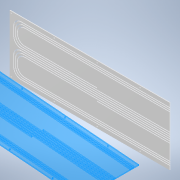
# Autodesk Inventor part: Part2
Saved by Autodesk Inventor 2021 (Build 250183000, 183)
## iProperties
Created: 2022-01-19
Part Number: Part2
Material: PVC-Piping
Document SubType Name: Modeling
Designer: avan411
Density: 1.4 g/cm^3
Appearance: Smooth - White
Author: avan411
Autodesk Inventor part; units mm, degrees
ref_plane "YZ Plane" through (0, 0, 0) normal (1, 0, 0) x (0, 1, 0)
ref_plane "XZ Plane" through (0, 0, 0) normal (0, 1, 0) x (-1, 0, 0)
ref_plane "XY Plane" through (0, 0, 0) normal (0, 0, 1) x (1, 0, 0)
sketch "Sketch1" plane through (0, 0, 0) normal (0, 0, 1) x (1, 0, 0)
  line L0 (97.5839, -88.8585) -> (97.5839, -84.5585) projected
  line L1 (97.5839, -88.8585) -> (532.0839, -88.8585) projected
  arc A0 (572.9339, -129.7085) -> (532.0839, -88.8585) centre (532.0839, -129.7085) ccw projected
  line L2 (572.9339, -129.7085) -> (572.9339, -137.9085) projected
  arc A1 (532.0839, -178.7585) -> (572.9339, -137.9085) centre (532.0839, -137.9085) ccw projected
  line L3 (532.0839, -178.7585) -> (-336.9161, -178.7585) projected
  arc A2 (-377.7661, -137.9085) -> (-336.9161, -178.7585) centre (-336.9161, -137.9085) ccw projected
  line L4 (-377.7661, -137.9085) -> (-377.7661, -118.2752) projected
  arc A3 (-336.9161, -77.4252) -> (-377.7661, -118.2752) centre (-336.9161, -118.2752) ccw projected
  line L5 (-336.9161, -77.4252) -> (543.3339, -77.4252) projected
  arc A4 (584.1839, -118.2752) -> (543.3339, -77.4252) centre (543.3339, -118.2752) ccw projected
  line L6 (584.1839, -118.2752) -> (584.1839, -148.6585) projected
  arc A5 (543.3339, -189.5085) -> (584.1839, -148.6585) centre (543.3339, -148.6585) ccw projected
  line L7 (543.3339, -189.5085) -> (-348.1661, -189.5085) projected
  arc A6 (-389.0161, -148.6585) -> (-348.1661, -189.5085) centre (-348.1661, -148.6585) ccw projected
  line L8 (-389.0161, -148.6585) -> (-389.0161, -106.8419) projected
  arc A7 (-348.1661, -65.9919) -> (-389.0161, -106.8419) centre (-348.1661, -106.8419) ccw projected
  line L9 (-348.1661, -65.9919) -> (554.5839, -65.9919) projected
  arc A8 (595.4339, -106.8419) -> (554.5839, -65.9919) centre (554.5839, -106.8419) ccw projected
  line L10 (595.4339, -106.8419) -> (595.4339, -159.4085) projected
  arc A9 (554.5839, -200.2585) -> (595.4339, -159.4085) centre (554.5839, -159.4085) ccw projected
  line L11 (554.5839, -200.2585) -> (-359.4161, -200.2585) projected
  arc A10 (-400.2661, -159.4085) -> (-359.4161, -200.2585) centre (-359.4161, -159.4085) ccw projected
  line L12 (-400.2661, -159.4085) -> (-400.2661, -95.4085) projected
  arc A11 (-359.4161, -54.5585) -> (-400.2661, -95.4085) centre (-359.4161, -95.4085) ccw projected
  line L13 (-359.4161, -54.5585) -> (554.5839, -54.5585) projected
  arc A12 (554.5839, -54.5585) -> (599.7339, -9.4085) centre (554.5839, -9.4085) ccw projected
  line L14 (599.7339, -9.4085) -> (599.7339, 54.5915) projected
  arc A13 (599.7339, 54.5915) -> (554.5839, 99.7415) centre (554.5839, 54.5915) ccw projected
  line L15 (554.5839, 99.7415) -> (-359.4161, 99.7415) projected
  arc A14 (-359.4161, 99.7415) -> (-404.5661, 54.5915) centre (-359.4161, 54.5915) ccw projected
  line L16 (-404.5661, 54.5915) -> (-404.5661, 2.0248) projected
  arc A15 (-404.5661, 2.0248) -> (-359.4161, -43.1252) centre (-359.4161, 2.0248) ccw projected
  line L17 (-359.4161, -43.1252) -> (543.3339, -43.1252) projected
  arc A16 (543.3339, -43.1252) -> (588.4839, 2.0248) centre (543.3339, 2.0248) ccw projected
  line L18 (588.4839, 2.0248) -> (588.4839, 43.8415) projected
  arc A17 (588.4839, 43.8415) -> (543.3339, 88.9915) centre (543.3339, 43.8415) ccw projected
  line L19 (543.3339, 88.9915) -> (-348.1661, 88.9915) projected
  arc A18 (-348.1661, 88.9915) -> (-393.3161, 43.8415) centre (-348.1661, 43.8415) ccw projected
  line L20 (-393.3161, 43.8415) -> (-393.3161, 13.4581) projected
  arc A19 (-393.3161, 13.4581) -> (-348.1661, -31.6919) centre (-348.1661, 13.4581) ccw projected
  line L21 (-348.1661, -31.6919) -> (532.0839, -31.6919) projected
  arc A20 (532.0839, -31.6919) -> (577.2339, 13.4581) centre (532.0839, 13.4581) ccw projected
  line L22 (577.2339, 13.4581) -> (577.2339, 33.0915) projected
  arc A21 (577.2339, 33.0915) -> (532.0839, 78.2415) centre (532.0839, 33.0915) ccw projected
  line L23 (532.0839, 78.2415) -> (-336.9161, 78.2415) projected
  arc A22 (-336.9161, 78.2415) -> (-382.0661, 33.0915) centre (-336.9161, 33.0915) ccw projected
  line L24 (-382.0661, 33.0915) -> (-382.0661, 24.8915) projected
  arc A23 (-382.0661, 24.8915) -> (-336.9161, -20.2585) centre (-336.9161, 24.8915) ccw projected
  line L25 (-336.9161, -20.2585) -> (97.5839, -20.2585) projected
  line L26 (97.5839, -15.9585) -> (97.5839, -20.2585) projected
  line L27 (-336.9161, -15.9585) -> (97.5839, -15.9585) projected
  arc A24 (-377.7661, 24.8915) -> (-336.9161, -15.9585) centre (-336.9161, 24.8915) ccw projected
  line L28 (-377.7661, 33.0915) -> (-377.7661, 24.8915) projected
  arc A25 (-336.9161, 73.9415) -> (-377.7661, 33.0915) centre (-336.9161, 33.0915) ccw projected
  line L29 (532.0839, 73.9415) -> (-336.9161, 73.9415) projected
  arc A26 (572.9339, 33.0915) -> (532.0839, 73.9415) centre (532.0839, 33.0915) ccw projected
  line L30 (572.9339, 13.4581) -> (572.9339, 33.0915) projected
  arc A27 (532.0839, -27.3919) -> (572.9339, 13.4581) centre (532.0839, 13.4581) ccw projected
  line L31 (-348.1661, -27.3919) -> (532.0839, -27.3919) projected
  arc A28 (-389.0161, 13.4581) -> (-348.1661, -27.3919) centre (-348.1661, 13.4581) ccw projected
  line L32 (-389.0161, 43.8415) -> (-389.0161, 13.4581) projected
  arc A29 (-348.1661, 84.6915) -> (-389.0161, 43.8415) centre (-348.1661, 43.8415) ccw projected
  line L33 (543.3339, 84.6915) -> (-348.1661, 84.6915) projected
  arc A30 (584.1839, 43.8415) -> (543.3339, 84.6915) centre (543.3339, 43.8415) ccw projected
  line L34 (584.1839, 2.0248) -> (584.1839, 43.8415) projected
  arc A31 (543.3339, -38.8252) -> (584.1839, 2.0248) centre (543.3339, 2.0248) ccw projected
  line L35 (-359.4161, -38.8252) -> (543.3339, -38.8252) projected
  arc A32 (-400.2661, 2.0248) -> (-359.4161, -38.8252) centre (-359.4161, 2.0248) ccw projected
  line L36 (-400.2661, 54.5915) -> (-400.2661, 2.0248) projected
  arc A33 (-359.4161, 95.4415) -> (-400.2661, 54.5915) centre (-359.4161, 54.5915) ccw projected
  line L37 (554.5839, 95.4415) -> (-359.4161, 95.4415) projected
  arc A34 (595.4339, 54.5915) -> (554.5839, 95.4415) centre (554.5839, 54.5915) ccw projected
  line L38 (595.4339, -9.4085) -> (595.4339, 54.5915) projected
  arc A35 (554.5839, -50.2585) -> (595.4339, -9.4085) centre (554.5839, -9.4085) ccw projected
  line L39 (-359.4161, -50.2585) -> (554.5839, -50.2585) projected
  arc A36 (-359.4161, -50.2585) -> (-404.5661, -95.4085) centre (-359.4161, -95.4085) ccw projected
  line L40 (-404.5661, -159.4085) -> (-404.5661, -95.4085) projected
  arc A37 (-404.5661, -159.4085) -> (-359.4161, -204.5585) centre (-359.4161, -159.4085) ccw projected
  line L41 (554.5839, -204.5585) -> (-359.4161, -204.5585) projected
  arc A38 (554.5839, -204.5585) -> (599.7339, -159.4085) centre (554.5839, -159.4085) ccw projected
  line L42 (599.7339, -106.8419) -> (599.7339, -159.4085) projected
  arc A39 (599.7339, -106.8419) -> (554.5839, -61.6919) centre (554.5839, -106.8419) ccw projected
  line L43 (-348.1661, -61.6919) -> (554.5839, -61.6919) projected
  arc A40 (-348.1661, -61.6919) -> (-393.3161, -106.8419) centre (-348.1661, -106.8419) ccw projected
  line L44 (-393.3161, -148.6585) -> (-393.3161, -106.8419) projected
  arc A41 (-393.3161, -148.6585) -> (-348.1661, -193.8085) centre (-348.1661, -148.6585) ccw projected
  line L45 (543.3339, -193.8085) -> (-348.1661, -193.8085) projected
  arc A42 (543.3339, -193.8085) -> (588.4839, -148.6585) centre (543.3339, -148.6585) ccw projected
  line L46 (588.4839, -118.2752) -> (588.4839, -148.6585) projected
  arc A43 (588.4839, -118.2752) -> (543.3339, -73.1252) centre (543.3339, -118.2752) ccw projected
  line L47 (-336.9161, -73.1252) -> (543.3339, -73.1252) projected
  arc A44 (-336.9161, -73.1252) -> (-382.0661, -118.2752) centre (-336.9161, -118.2752) ccw projected
  line L48 (-382.0661, -137.9085) -> (-382.0661, -118.2752) projected
  arc A45 (-382.0661, -137.9085) -> (-336.9161, -183.0585) centre (-336.9161, -137.9085) ccw projected
  line L49 (532.0839, -183.0585) -> (-336.9161, -183.0585) projected
  arc A46 (532.0839, -183.0585) -> (577.2339, -137.9085) centre (532.0839, -137.9085) ccw projected
  line L50 (577.2339, -129.7085) -> (577.2339, -137.9085) projected
  arc A47 (577.2339, -129.7085) -> (532.0839, -84.5585) centre (532.0839, -129.7085) ccw projected
  line L51 (97.5839, -84.5585) -> (532.0839, -84.5585) projected
  line L52 (97.5839, -20.2585) -> (97.5839, -84.5585) construction
  line L53 (97.5839, -52.4085) -> (22.8086, -52.4085)
  line L54 (-427.4161, 122.5915) -> (532.0839, 122.5915)
  line L55 (532.0839, 122.5915) -> (532.0839, -227.4085)
  line L56 (532.0839, -227.4085) -> (-427.4161, -227.4085)
  line L57 (-427.4161, -227.4085) -> (-427.4161, 122.5915)
  circle A48 centre (355.0839, -217.4085) radius 3 projected
  circle A49 centre (97.5839, -217.4085) radius 3 projected
  circle A50 centre (-159.9161, -217.4085) radius 3 projected
  circle A51 centre (-417.4161, -217.4085) radius 3 projected
  circle A52 centre (-417.4161, 112.5915) radius 3 projected
  circle A53 centre (-159.9161, 112.5915) radius 3 projected
  circle A54 centre (355.0839, 112.5915) radius 3 projected
  circle A55 centre (97.5839, 112.5915) radius 3 projected
  circle A56 centre (355.0839, -217.4085) radius 3
  circle A57 centre (97.5839, -217.4085) radius 3
  circle A58 centre (-159.9161, -217.4085) radius 3
  circle A59 centre (-417.4161, -217.4085) radius 3
  circle A60 centre (-417.4161, 112.5915) radius 3
  circle A61 centre (-159.9161, 112.5915) radius 3
  circle A62 centre (97.5839, 112.5915) radius 3
  circle A63 centre (355.0839, 112.5915) radius 3
  point P0 (0, 0)
  point P1 (-336.9161, -31.6919)
  point P2 (-336.9161, -38.8252)
  point P3 (-336.9161, 84.6915)
  point P4 (-336.9161, -43.1252)
  point P5 (-336.9161, -50.2585)
  point P6 (-336.9161, 95.4415)
  point P7 (-336.9161, 88.9915)
  point P8 (-336.9161, -65.9919)
  point P9 (-336.9161, -193.8085)
  point P10 (-336.9161, -200.2585)
  point P11 (-336.9161, -189.5085)
  point P12 (-336.9161, -178.7585)
  point P13 (-336.9161, -54.5585)
  point P14 (-336.9161, -61.6919)
  point P15 (-336.9161, -204.5585)
  point P16 (-336.9161, 99.7415)
  point P17 (-336.9161, -27.3919)
  point P18 (532.0839, -38.8252)
  point P19 (532.0839, 84.6915)
  point P20 (532.0839, -189.5085)
  point P21 (532.0839, -193.8085)
  point P22 (532.0839, -73.1252)
  point P23 (532.0839, -77.4252)
  point P24 (532.0839, -54.5585)
  point P25 (532.0839, -50.2585)
  point P26 (532.0839, -204.5585)
  point P27 (532.0839, -200.2585)
  point P28 (532.0839, -43.1252)
  point P29 (532.0839, 95.4415)
  point P30 (532.0839, 88.9915)
  point P31 (532.0839, 99.7415)
  point P32 (532.0839, -65.9919)
  point P33 (532.0839, -61.6919)
  dimension "d6" = 350
  dimension "d7" = 175
  dimension "d10" = 525
  dimension "d11" = 0
  constraints: 8 centre point, 8 coincident, 8 concentric, 8 end point, 2 horizontal, 2 parallel, 1 midpoint, 1 perpendicular, 6 other
  measures "d6" distance between parallel lines of L56 L54
  measures "d7" distance from line of L53.start L56
extrude "Extrusion4" add sketch "Sketch1" along normal blind 5 contours L1 L55 L3 A2 L4 A3 L5 L51 L0 | L55 L7 A6 L8 A7 L9 L47 A44 L48 A45 L49 | L55 L11 A10 L12 A11 L13 L43 A40 L44 A41 L45 | L55 L56 L57 L54 L15 A14 L16 A15 L17 L39 A36 L40 A37 L41 | L35 A32 L36 A33 L37 L55 L19 A18 L20 A19 L21 | L31 A28 L32 A29 L33 L55 L23 A22 L24 A23 L25 L26 L27 A24 L28 A25 L29
body "Solid4"
